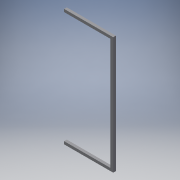
# Autodesk Inventor part: Drop Loop
Saved by Autodesk Inventor 2018 (Build 220112000, 112)
## iProperties
Created: 2018-01-29
Part Number: Drop Loop
Material: Generic
Document SubType Name: Modeling
Designer: Apple
Density: 1 g/cm^3
Appearance: Default
Author: Apple
Autodesk Inventor part; units mm, degrees
ref_plane "YZ Plane" through (0, 0, 0) normal (1, 0, 0) x (0, 1, 0)
ref_plane "XZ Plane" through (0, 0, 0) normal (0, 1, 0) x (-1, 0, 0)
ref_plane "XY Plane" through (0, 0, 0) normal (0, 0, 1) x (1, 0, 0)
sketch "Sketch1" plane through (0, 0, 0) normal (0, 0, 1) x (1, 0, 0)
  line L0 (0, 0) -> (66.675, 0) projected
  line L1 (66.675, 0) -> (66.675, 685.8) projected
  line L2 (0, 685.8) -> (66.675, 685.8) projected
  line L3 (0, 0) -> (0, 685.8) projected
  line L4 (0, 69.85) -> (228.6, 69.85)
  line L5 (228.6, 69.85) -> (228.6, 615.95)
  line L6 (228.6, 615.95) -> (0, 615.95)
  line L7 (0, 82.55) -> (215.9, 82.55)
  line L8 (215.9, 82.55) -> (215.9, 603.25)
  line L9 (215.9, 603.25) -> (0, 603.25)
  line L10 (0, 69.85) -> (0, 82.55)
  line L11 (0, 603.25) -> (0, 615.95)
  point P0 (228.6, 342.9)
  point P1 (0, 342.9)
  dimension "d0" = 546.1
  dimension "d1" = 228.6
  dimension "d2" = 12.7
  constraints: 16 end point, 4 perpendicular, 2 midpoint, 2 point on line, 1 collinear, 1 horizontal, 1 horizontal alignment, 1 vertical, 2 other
  measures "d0" distance of L4.end L5.end
  measures "d1" distance of L4.start L4.end
  measures "d2" distance between parallel lines of L4 L7
extrude "Extrusion1" add sketch "Sketch1" along normal blind 12.7 contours L3 L7 L1 L4 | L1 L7 L8 L9 L6 L5 L4 | L3 L6 L1 L9
body "Solid1"
